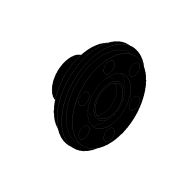
# Autodesk Inventor part: Mounting Plate
Saved by Autodesk Inventor 2020 (Build 240168000, 168)
## iProperties
Created: 2021-06-29
Part Number: Mounting Plate
Material: Generic
Document SubType Name: Modeling
Designer: Coy
Density: 1 g/cm^3
Appearance: Anodized - Black
Author: Coy
Autodesk Inventor part; units mm, degrees
ref_plane "YZ Plane" through (0, 0, 0) normal (1, 0, 0) x (0, 1, 0)
ref_plane "XZ Plane" through (0, 0, 0) normal (0, 1, 0) x (-1, 0, 0)
ref_plane "XY Plane" through (0, 0, 0) normal (0, 0, 1) x (1, 0, 0)
sketch "Sketch1" plane through (0, 0, 0) normal (1, 0, 0) x (0, 1, 0)
  circle A0 centre (0, 0) radius 24
  circle A1 centre (0, 0) radius 14
  circle A2 centre (0, 0) radius 19 construction
  circle A3 centre (19, 0) radius 3.5
  circle A4 centre (9.5, 16.4545) radius 3.5
  circle A5 centre (-9.5, 16.4545) radius 3.5
  circle A6 centre (-19, 0) radius 3.5
  circle A7 centre (-9.5, -16.4545) radius 3.5
  circle A8 centre (9.5, -16.4545) radius 3.5
  circle A9 centre (0, 0) radius 10
  circle A10 centre (0, 0) radius 9
  dimension "d0" = 48
  dimension "d1" = 10
  dimension "d2" = 5
  dimension "d3" = 7
  dimension "d6" = 360
  dimension "d8" = 20
  dimension "d9" = 1
  constraints: 10 centre point, 2 coincident, 1 horizontal alignment, 15 other
  measures "d0" diameter of A0
  measures "d1" radial gap between concentric circles of A0 A1
  measures "d3" diameter of A3
  measures "d8" diameter of A9
  measures "d9" radial gap between concentric circles of A9 A10
extrude "Extrusion1" add sketch "Sketch1" against normal blind 4
sketch "Sketch2" plane through (-4, 0, 0) normal (-1, 0, 0) x (0, 0, 1)
  circle A0 centre (0, 0) radius 24 projected
  circle A1 centre (-16.4545, 9.5) radius 3.5 projected
  circle A2 centre (16.4545, 9.5) radius 3.5 projected
  circle A3 centre (0, 19) radius 3.5 projected
  circle A4 centre (-16.4545, -9.5) radius 3.5 projected
  circle A5 centre (0, -19) radius 3.5 projected
  circle A6 centre (16.4545, -9.5) radius 3.5 projected
  circle A7 centre (0, 0) radius 14 projected
  circle A8 centre (0, 0) radius 27
  dimension "d12" = 3
  constraints: 1 centre point
  measures "d12" radial gap between concentric circles of A0 A8
extrude "Extrusion2" add sketch "Sketch2" along normal blind 3 contours A0 | A7 | A8
sketch "Sketch3" plane through (-7, 0, 0) normal (-1, 0, 0) x (0, 0, 1)
  circle A0 centre (0, 0) radius 27 projected
  circle A1 centre (0, 19) radius 3.5 projected
  circle A2 centre (-16.4545, -9.5) radius 3.5 projected
  circle A3 centre (-16.4545, 9.5) radius 3.5 projected
  circle A4 centre (16.4545, 9.5) radius 3.5 projected
  circle A5 centre (0, -19) radius 3.5 projected
  circle A6 centre (16.4545, -9.5) radius 3.5 projected
  circle A7 centre (0, 0) radius 24 projected
extrude "Extrusion3" add sketch "Sketch3" along normal blind 3 contours A7
sketch "Sketch4" plane through (-10, 0, 0) normal (-1, 0, 0) x (0, 0, 1)
  circle A0 centre (0, 0) radius 24 projected
extrude "Extrusion4" add sketch "Sketch4" along normal blind 2
sketch "Sketch5" plane through (-12, 0, 0) normal (-1, 0, 0) x (0, 0, 1)
  circle A0 centre (0, 0) radius 12.5
  dimension "d19" = 25
  constraints: 1 centre point, 1 coincident
  measures "d19" diameter of A0
extrude "Extrusion5" add sketch "Sketch5" along normal blind 7
chamfer "Chamfer1" distance 7 angle 2 1 edges at (-19, 0, -12.5) measured on face at (-18.5, 0, -12.5)
sketch "Sketch6" plane through (-19, 0, 0) normal (-1, 0, 0) x (0, 0, 1)
  circle A0 centre (0, 0) radius 12.5 construction
  circle A1 centre (0, 0) radius 12.2556 projected
  line L0 (0, 0) -> (0, 14.9794) construction
  arc A2 (0.2, 12.4968) -> (-0.2, 12.4968) centre (0, 12.5) ccw
  line L1 (0.1961, 12.254) -> (0.2, 12.4984)
  line L2 (-0.1961, 12.254) -> (-0.2, 12.4984)
  line L3 (-10.7103, 5.9572) -> (-10.9239, 6.076)
  arc A3 (-10.7226, 6.4216) -> (-10.9225, 6.0752) centre (-10.8253, 6.25) ccw
  line L4 (-10.5142, 6.2968) -> (-10.7239, 6.4224)
  line L5 (-10.5142, -6.2968) -> (-10.7239, -6.4224)
  arc A4 (-10.9225, -6.0752) -> (-10.7226, -6.4216) centre (-10.8253, -6.25) ccw
  line L6 (-10.7103, -5.9572) -> (-10.9239, -6.076)
  line L7 (0.1961, -12.254) -> (0.2, -12.4984)
  arc A5 (-0.2, -12.4968) -> (0.2, -12.4968) centre (0, -12.5) ccw
  line L8 (-0.1961, -12.254) -> (-0.2, -12.4984)
  line L9 (10.7103, -5.9572) -> (10.9239, -6.076)
  arc A6 (10.7226, -6.4216) -> (10.9225, -6.0752) centre (10.8253, -6.25) ccw
  line L10 (10.5142, -6.2968) -> (10.7239, -6.4224)
  line L11 (10.5142, 6.2968) -> (10.7239, 6.4224)
  arc A7 (10.9225, 6.0752) -> (10.7226, 6.4216) centre (10.8253, 6.25) ccw
  line L12 (10.7103, 5.9572) -> (10.9239, 6.076)
  dimension "d25" = 0.4
  dimension "d28" = 360
  constraints: 26 end point, 17 point on circle, 13 point on line, 6 centre point, 2 line through centre, 2 tangent, 1 vertical, 61 other
  measures "d25" diameter of A2
extrude "Extrusion6" add sketch "Sketch6" against normal blind 7 contours A1 L11 A7 L12 | L9 A6 L10 A1 | A1 L2 A2 L1 | L7 A5 L8 A1 | A1 L3 A3 L4 | L5 A4 L6 A1
sketch "Sketch7" plane through (-19, 0, 0) normal (-1, 0, 0) x (0, 0, 1)
  line L0 (-0.2, 12.4968) -> (-0.1961, 12.254) projected
  circle A0 centre (0, 0) radius 12.2556
  constraints: 1 coincident, 3 other
extrude "Extrusion7" add sketch "Sketch7" along normal blind 1
sketch "Sketch8" plane through (-20, 0, 0) normal (-1, 0, 0) x (0, 0, 1)
  circle A0 centre (0, 0) radius 12.2556 projected
  line L0 (0, 0) -> (0, 17.9817) construction
  circle A1 centre (0, 0) radius 11.2556
  circle A2 centre (0, 0) radius 9.0556 construction
  arc A3 (-1.0443, 9.9965) -> (1.0443, 9.9965) centre (0, 10.1056) ccw
  line L1 (1.0548, 10.0965) -> (1.0443, 9.9965)
  line L2 (-1.0548, 10.0965) -> (-1.0443, 9.9965)
  arc A4 (-1.0548, 10.0965) -> (-2.315, 11.0149) centre (-2.0991, 9.9874) ccw
  arc A5 (2.315, 11.0149) -> (1.0548, 10.0965) centre (2.0991, 9.9874) ccw
  arc A6 (-5.0702, 8.7946) -> (-6.5951, 9.121) centre (-5.9798, 8.2701) ccw
  line L3 (-5.0702, 8.7946) -> (-5.02, 8.7075)
  arc A7 (-5.02, 8.7075) -> (-3.1119, 9.557) centre (-4.1103, 9.2319) ccw
  line L4 (-3.143, 9.6526) -> (-3.1119, 9.557)
  arc A8 (-2.3653, 11.0042) -> (-3.143, 9.6526) centre (-2.1446, 9.9777) ccw
  arc A9 (-8.2089, 5.972) -> (-9.7347, 5.65) centre (-8.8266, 5.1229) ccw
  line L5 (-8.2089, 5.972) -> (-8.1276, 5.9129)
  arc A10 (-8.1276, 5.9129) -> (-6.73, 7.465) centre (-7.5099, 6.7619) ccw
  line L6 (-6.7974, 7.5397) -> (-6.73, 7.465)
  arc A11 (-6.6366, 9.0908) -> (-6.7974, 7.5397) centre (-6.0175, 8.2428) ccw
  arc A12 (-9.9282, 2.1168) -> (-11.1912, 1.2021) centre (-10.1472, 1.0899) ccw
  line L7 (-9.9282, 2.1168) -> (-9.8299, 2.0959)
  arc A13 (-9.8299, 2.0959) -> (-9.1845, 4.0823) centre (-9.611, 3.1228) ccw
  line L8 (-9.2764, 4.1231) -> (-9.1845, 4.0823)
  arc A14 (-9.7604, 5.6055) -> (-9.2764, 4.1231) centre (-8.8499, 5.0826) ccw
  arc A15 (-9.9309, -2.1044) -> (-10.7126, -3.4537) centre (-9.7132, -3.1315) ccw
  line L9 (-9.9309, -2.1044) -> (-9.8325, -2.0835)
  arc A16 (-9.8325, -2.0835) -> (-10.0509, -0.0063) centre (-10.0502, -1.0563) ccw
  line L10 (-10.1514, -0.0064) -> (-10.0509, -0.0063)
  arc A17 (-11.1965, 1.151) -> (-10.1514, -0.0064) centre (-10.1521, 1.0436) ccw
  arc A18 (-8.2164, -5.9617) -> (-8.3817, -7.5123) centre (-7.5998, -6.8115) ccw
  line L11 (-8.2164, -5.9617) -> (-8.135, -5.9026)
  arc A19 (-8.135, -5.9026) -> (-9.1793, -4.0938) centre (-8.7517, -5.0528) ccw
  line L12 (-9.2712, -4.1348) -> (-9.1793, -4.0938)
  arc A20 (-10.6967, -3.5026) -> (-9.2712, -4.1348) centre (-9.6988, -3.1758) ccw
  arc A21 (-5.0812, -8.7882) -> (-4.6015, -10.272) centre (-4.1722, -9.3137) ccw
  line L13 (-5.0812, -8.7882) -> (-5.0309, -8.7011)
  arc A22 (-5.0309, -8.7011) -> (-6.7206, -7.4735) centre (-5.9399, -8.1756) ccw
  line L14 (-6.7879, -7.5482) -> (-6.7206, -7.4735)
  arc A23 (-8.3473, -7.5505) -> (-6.7879, -7.5482) centre (-7.5686, -6.8461) ccw
  arc A24 (-1.0675, -10.0951) -> (-0.0257, -11.2555) centre (-0.0233, -10.2055) ccw
  line L15 (-1.0675, -10.0951) -> (-1.0569, -9.9951)
  arc A25 (-1.0569, -9.9951) -> (-3.0999, -9.5609) centre (-2.1011, -9.8847) ccw
  line L16 (-3.1309, -9.6565) -> (-3.0999, -9.5609)
  arc A26 (-4.5546, -10.2929) -> (-3.1309, -9.6565) centre (-4.1297, -9.3327) ccw
  arc A27 (3.1309, -9.6565) -> (4.5546, -10.2929) centre (4.1297, -9.3327) ccw
  line L17 (3.1309, -9.6565) -> (3.0999, -9.5609)
  arc A28 (3.0999, -9.5609) -> (1.0569, -9.9951) centre (2.1011, -9.8847) ccw
  line L18 (1.0675, -10.0951) -> (1.0569, -9.9951)
  arc A29 (0.0257, -11.2555) -> (1.0675, -10.0951) centre (0.0233, -10.2055) ccw
  arc A30 (6.7879, -7.5482) -> (8.3473, -7.5505) centre (7.5686, -6.8461) ccw
  line L19 (6.7879, -7.5482) -> (6.7206, -7.4735)
  arc A31 (6.7206, -7.4735) -> (5.0309, -8.7011) centre (5.9399, -8.1756) ccw
  line L20 (5.0812, -8.7882) -> (5.0309, -8.7011)
  arc A32 (4.6015, -10.272) -> (5.0812, -8.7882) centre (4.1722, -9.3137) ccw
  arc A33 (9.2712, -4.1348) -> (10.6967, -3.5026) centre (9.6988, -3.1758) ccw
  line L21 (9.2712, -4.1348) -> (9.1793, -4.0938)
  arc A34 (9.1793, -4.0938) -> (8.135, -5.9026) centre (8.7517, -5.0528) ccw
  line L22 (8.2164, -5.9617) -> (8.135, -5.9026)
  arc A35 (8.3817, -7.5123) -> (8.2164, -5.9617) centre (7.5998, -6.8115) ccw
  arc A36 (10.1514, -0.0064) -> (11.1965, 1.151) centre (10.1521, 1.0436) ccw
  line L23 (10.1514, -0.0064) -> (10.0509, -0.0063)
  arc A37 (10.0509, -0.0063) -> (9.8325, -2.0835) centre (10.0502, -1.0563) ccw
  line L24 (9.9309, -2.1044) -> (9.8325, -2.0835)
  arc A38 (10.7126, -3.4537) -> (9.9309, -2.1044) centre (9.7132, -3.1315) ccw
  arc A39 (9.2764, 4.1231) -> (9.7604, 5.6055) centre (8.8499, 5.0826) ccw
  line L25 (9.2764, 4.1231) -> (9.1845, 4.0823)
  arc A40 (9.1845, 4.0823) -> (9.8299, 2.0959) centre (9.611, 3.1228) ccw
  line L26 (9.9282, 2.1168) -> (9.8299, 2.0959)
  arc A41 (11.1912, 1.2021) -> (9.9282, 2.1168) centre (10.1472, 1.0899) ccw
  arc A42 (6.7974, 7.5397) -> (6.6366, 9.0908) centre (6.0175, 8.2428) ccw
  line L27 (6.7974, 7.5397) -> (6.73, 7.465)
  arc A43 (6.73, 7.465) -> (8.1276, 5.9129) centre (7.5099, 6.7619) ccw
  line L28 (8.2089, 5.972) -> (8.1276, 5.9129)
  arc A44 (9.7347, 5.65) -> (8.2089, 5.972) centre (8.8266, 5.1229) ccw
  arc A45 (3.143, 9.6526) -> (2.3653, 11.0042) centre (2.1446, 9.9777) ccw
  line L29 (3.143, 9.6526) -> (3.1119, 9.557)
  arc A46 (3.1119, 9.557) -> (5.02, 8.7075) centre (4.1103, 9.2319) ccw
  line L30 (5.0702, 8.7946) -> (5.02, 8.7075)
  arc A47 (6.5951, 9.121) -> (5.0702, 8.7946) centre (5.9798, 8.2701) ccw
  point P0 (4.5546, -10.2929)
  point P1 (-0.0257, -11.2555)
  point P2 (-4.5546, -10.2929)
  point P3 (-11.1965, 1.151)
  point P4 (-9.7604, 5.6055)
  point P5 (-9.7347, 5.65)
  point P6 (6.6366, 9.0908)
  point P7 (9.7347, 5.65)
  point P8 (11.1965, 1.151)
  dimension "d35" = 1
  dimension "d36" = 2.2
  dimension "d37" = 2.1
  dimension "d38" = 2.1
  dimension "d39" = 2.1
  dimension "d42" = 360
  constraints: 90 point on circle, 62 end point, 46 centre point, 5 tangent, 1 point on line, 1 vertical, 219 other
  measures "d37" diameter of A3
  measures "d38" diameter of A4
  measures "d39" diameter of A5
extrude "Extrusion8" add sketch "Sketch8" along normal blind 5 contours A0 | A1 A38 L24 A37 L23 A36 | A41 L26 A40 L25 A39 A1 | A1 A35 L22 A34 L21 A33 | A44 L28 A43 L27 A42 A1 | A1 A32 L20 A31 L19 A30 | A47 L30 A46 L29 A45 A1 | A1 A29 L18 A28 L17 A27 | A5 L1 A3 L2 A4 A1 | A1 A26 L16 A25 L15 A24 | A8 L4 A7 L3 A6 A1 | A1 A23 L14 A22 L13 A21 | A11 L6 A10 L5 A9 A1 | A1 A20 L12 A19 L11 A18 | A14 L8 A13 L7 A12 A1 | A1 A17 L10 A16 L9 A15
equation "\"d38\" = d37"
equation "\"d39\" = d37"
body "Solid1"
